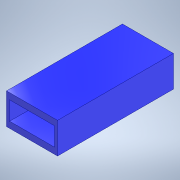
# Autodesk Inventor part: Electronics Lid
Saved by Autodesk Inventor 2022 (Build 260153000, 153)
## iProperties
Created: 2022-08-13
Part Number: Electronics Lid
Material: Generic
Document SubType Name: Modeling
Designer: Nick
Density: 1 g/cm^3
Appearance: Blue - Wall Paint - Glossy
Author: Nick
Autodesk Inventor part; units mm, degrees
ref_plane "YZ Plane" through (0, 0, 0) normal (1, 0, 0) x (0, 1, 0)
ref_plane "XZ Plane" through (0, 0, 0) normal (0, 1, 0) x (-1, 0, 0)
ref_plane "XY Plane" through (0, 0, 0) normal (0, 0, 1) x (1, 0, 0)
sketch "Sketch1" plane through (0, 0, 0) normal (0, 0, 1) x (1, 0, 0)
  line L0 (0, 0) -> (33, 0)
  line L1 (33, 0) -> (33, 4)
  line L2 (33, 4) -> (0, 4)
  line L3 (0, 4) -> (0, 0)
  line L4 (0, 20) -> (33, 20)
  line L5 (33, 20) -> (33, 16)
  line L6 (33, 16) -> (0, 16)
  line L7 (0, 16) -> (0, 20)
  line L8 (33, 16) -> (31, 16)
  line L9 (31, 16) -> (31, 4)
  line L10 (31, 4) -> (33, 4)
  line L11 (33, 4) -> (33, 16)
  line L12 (0, 16) -> (2, 16)
  line L13 (2, 16) -> (2, 4)
  line L14 (2, 4) -> (0, 4)
  line L15 (0, 4) -> (0, 16)
  point P0 (2, 16)
  point P1 (31, 4)
  point P2 (2, 4)
  dimension "d0" = 4
  dimension "d1" = 12
  dimension "d2" = 29
  dimension "d5" = 2
  dimension "d6" = 2
  constraints: 32 end point, 8 parallel, 4 horizontal, 4 perpendicular, 1 collinear
  measures "d0" distance of L0.end L1.end
  measures "d1" distance of L8.end L9.end
  measures "d2" distance between parallel lines of L9 L13
  measures "d5" distance between parallel lines of L11 L9
  measures "d6" distance between parallel lines of L15 L13
extrude "Extrusion1" add sketch "Sketch1" along normal blind 75 contours L3 L2 L1 L0 | L15 L6 L13 L2 | L2 L9 L6 L11 | L7 L4 L5 L6
body "Solid1"
